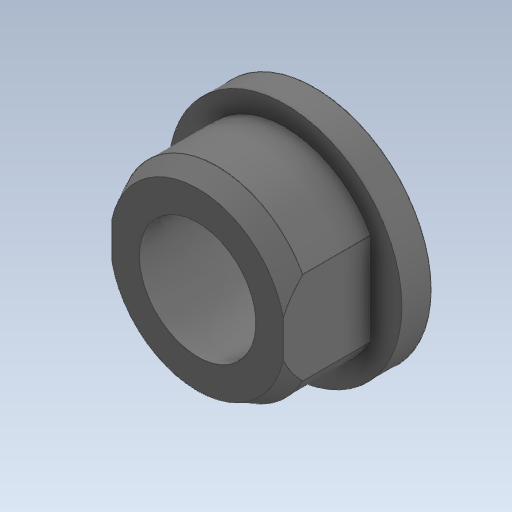
# Autodesk Inventor part: LED-0606
Saved by Autodesk Inventor 2020.4 (Build 244396000, 396)
## iProperties
Part Number: LED-0606
Material: アセタール樹脂、黒
Document SubType Name: Modeling
Designer: Masato Kubotera
Density: 1.3613 g/cm^3
Appearance: 灰色
Description: ReadyMade
Mass: 0.45 g
Surface Area: 4.68851 cm^2
Volume: 0.330566 cm^3
Catalog Web Link: https://jp.misumi-ec.com/vona2/detail/221000090992/?HissuCode=LED-0606
Author: Masato Kubotera
Autodesk Inventor part; units mm, degrees
ref_plane "YZ Plane" through (0, 0, 0) normal (1, 0, 0) x (0, 1, 0)
ref_plane "XZ Plane" through (0, 0, 0) normal (0, 1, 0) x (-1, 0, 0)
ref_plane "XY Plane" through (0, 0, 0) normal (0, 0, 1) x (1, 0, 0)
sketch "スケッチ1" plane through (0, 0, 0) normal (0, 1, 0) x (-1, 0, 0)
  line L0 (3, 0) -> (6, 0)
  line L1 (6, 0) -> (6, 1.5)
  line L2 (6, 1.5) -> (5, 1.5)
  line L3 (5, 1.5) -> (5, 5)
  line L4 (4.5, 6) -> (3, 6)
  line L5 (3, 6) -> (3, 0)
  line L6 (5, 5) -> (4.5, 6)
  line L7 (0, -1.2) -> (0, 7.2) projected
  point P0 (0, 0)
  point P1 (3, 6)
  dimension "d5" = 1.5
  dimension "d9" = 1
  dimension "d10" = 0.5
  dimension "d17" = 10
  dimension "d18" = 12
  dimension "d19" = 6
  dimension "d20" = 6
  constraints: 14 end point, 4 perpendicular, 1 horizontal, 1 parallel, 1 point on line
  measures "d5" distance of L0.end L1.end
  measures "d9" vertical distance of L3.end L4.start
  measures "d10" horizontal distance of L4.start L3.end
  measures "d17" diameter of L3.end L7
  measures "d18" diameter of L0.end L7
  measures "d19" distance of L4.end L0.start
  measures "d20" diameter of L5 L7
revolve "回転1" add sketch "スケッチ1" angle 360 about axis through (0, 0, -10) along (0, 0, 1)
sketch "スケッチ2" plane through (0, 0, 6) normal (0, 0, 1) x (1, 0, 0)
  line L0 (4.4, -2.3749) -> (-4.4, -2.3749)
  line L1 (-4.4, -2.3749) -> (-4.4, 2.3749)
  line L2 (-4.4, 2.3749) -> (4.4, 2.3749)
  line L3 (4.4, 2.3749) -> (4.4, -2.3749)
  line L4 (4.4, -2.3749) -> (-4.4, 2.3749) construction
  line L5 (-4.4, -2.3749) -> (4.4, 2.3749) construction
  circle A0 centre (0, 0) radius 5
  point P0 (0, 0)
  dimension "d12" = 10
  dimension "d11" = 8.8
  constraints: 12 end point, 2 midpoint, 2 parallel, 1 coincident, 1 horizontal, 1 perpendicular, 3 other
  measures "d11" distance of L1.end L2.end
extrude "押し出し1" cut sketch "スケッチ2" against normal up to surface (4.5 mm away) contours L3 A0 | A0 L1
